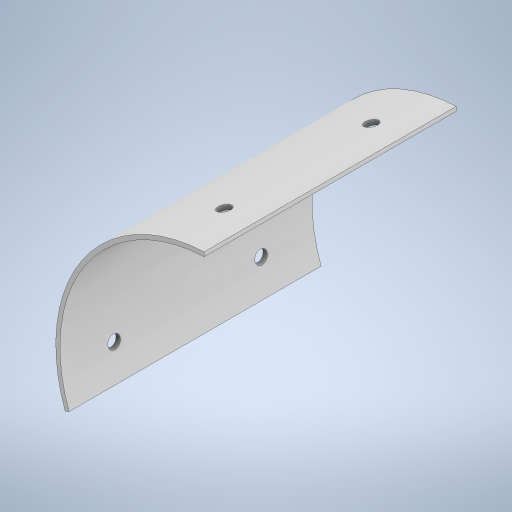
# Autodesk Inventor part: Electronics Door
Saved by Autodesk Inventor 2024 (Build 280153000, 153)
## iProperties
Created: 2024-04-23
Part Number: Electronics Door
Material: Generic
Document SubType Name: Modeling
Designer: auror
Density: 1 g/cm^3
Appearance: Default
Author: auror
Autodesk Inventor part; units mm, degrees
ref_plane "YZ Plane" through (0, 0, 0) normal (1, 0, 0) x (0, 1, 0)
ref_plane "XZ Plane" through (0, 0, 0) normal (0, 1, 0) x (-1, 0, 0)
ref_plane "XY Plane" through (0, 0, 0) normal (0, 0, 1) x (1, 0, 0)
sketch "Sketch1" plane through (0, 0, 0) normal (0, 0, 1) x (1, 0, 0)
  line L0 (0, 39.5237) -> (0, -43.4686) construction
  line L1 (-45.3066, 0) -> (2.8066, 0) construction
  line L2 (-11.1644, 34.052) -> (-34, 0) construction
  line L3 (2.8066, 0) -> (-40.0076, 0) construction
  line L4 (16.398, -33.1268) -> (-15.7593, 45.2513) construction
  line L5 (2.8066, 0) -> (-40.7672, -15.8596) construction
  arc A0 (-10.7848, 33.1268) -> (-33, 0) centre (2.8066, 0) ccw
  arc A1 (-11.1644, 34.052) -> (-34, 0) centre (2.8066, 0) ccw
  line L6 (1.3246, 36.7767) -> (1.3246, 35.7759)
  line L7 (-33, 0) -> (-34, 0)
  arc A2 (1.3246, 35.7759) -> (-10.7848, 33.1268) centre (2.8066, 0) ccw
  arc A3 (-33, 0) -> (-30.8406, -12.2466) centre (2.8066, 0) ccw
  arc A4 (1.3246, 36.7767) -> (-11.1644, 34.052) centre (2.8066, 0) ccw
  arc A5 (-34, 0) -> (-31.7803, -12.5886) centre (2.8066, 0) ccw
  line L8 (-34, 0) -> (-33, 0) construction
  line L9 (-31.7803, -12.5886) -> (-30.8406, -12.2466)
  line L10 (-34, 0) -> (-33, 0)
  line L11 (-11.1644, 34.052) -> (-10.7848, 33.1268)
  line L12 (2.8066, 0) -> (0.7848, 50.1716) construction
  point P0 (0, 0)
  point P1 (0, 35.5701)
  point P2 (-35.7519, 0.9163)
  dimension "d17" = 41
  dimension "d18" = 0
  dimension "d19" = 0
  dimension "d22" = 20
  dimension "d26" = 0
  dimension "d27" = 0
  dimension "d28" = 0
  dimension "d29" = 0
  dimension "d73" = 0
  dimension "d74" = 20
  constraints: 26 end point, 14 point on circle, 11 point on line, 6 centre point, 4 coincident, 4 collinear, 3 vertical, 1 horizontal, 1 perpendicular
  measures "d17" distance of L2.start L2.end
  measures "d18" distance from line of L1 L2.end
  measures "d19" distance from line of L2.end L3
  measures "d22" angle of L5 L1
  measures "d26" distance of L2.end L8.start
  measures "d27" distance of L7.start L8.end
  measures "d28" distance of L2.start L11.start
  measures "d29" distance of A0.start L11.end
  measures "d73" distance from line of L6.start L12
  measures "d74" angle of L12 L4
extrude "Extrusion2" add sketch "Sketch1" along normal blind 60 contours L11 A4 L6 A2
extrude "Extrusion3" add sketch "Sketch1" along normal blind 60 fills toward (-27.7211, 20.4722) open curves A1 L7 A0
extrude "Extrusion4" add sketch "Sketch1" along normal blind 60 contours A3 L9 A5 L7
ref_plane "Work Plane2" through (-11.1644, 34.052, 0) normal (-0.3795786, 0.9251595, 0) x (-0.9251595, -0.3795786, 0)
sketch "Sketch3" plane through (-11.1644, 34.052, 0) normal (-0.3795786, 0.9251595, 0) x (-0.9251595, -0.3795786, 0)
  line L0 (36.7767, 0) -> (-12.5886, 0) projected
  line L1 (-0.001, 0) -> (-0.001, 27.4188)
  point P0 (2.5965, 0)
  point P1 (-5.001, 12.5)
  dimension "d37" = 12.5
  dimension "d38" = 5
  constraints: 2 end point, 2 vertical, 1 point on line
  measures "d37" distance from line of L0 point (-5.001, 12.5)
  measures "d38" distance from line of L1 point (-5.001, 12.5)
hole "Hole1" at (-6.5377, 35.9502, 12.5) direction (0.3795786, -0.9251595, 0) diameter 2 end through all counterbore diameter 3 counterbore depth 10
sketch "Sketch4" plane through (-11.1644, 34.052, 0) normal (-0.3795786, 0.9251595, 0) x (-0.9251595, -0.3795786, 0)
  line L0 (36.7767, 60) -> (-12.5886, 60) projected
  line L1 (-0.0225, 60) -> (-0.0225, 43.6273)
  point P0 (2.5965, 0)
  point P1 (-5.0225, 47.5)
  dimension "d46" = 12.5
  dimension "d47" = 5
  constraints: 2 end point, 2 vertical, 1 point on line
  measures "d46" distance from line of L0 point (-5.022, 47.5)
  measures "d47" distance from line of L1 point (-5.022, 47.5)
hole "Hole2" at (-6.5178, 35.9584, 47.5) direction (0.3795786, -0.9251595, 0) diameter 2 end through all counterbore diameter 3 counterbore depth 10
ref_plane "Work Plane3" through (-34, 0, 0) normal (-1, 0, 0) x (0, -1, 0)
sketch "Sketch5" plane through (-34, 0, 0) normal (-1, 0, 0) x (0, -1, 0)
  line L0 (12.5886, 0) -> (-36.7767, 0) projected
  line L1 (0, 0) -> (0, 12.4269)
  point P0 (5, 12.5)
  dimension "d55" = 12.5
  dimension "d56" = 5
  constraints: 2 end point, 2 vertical
  measures "d55" distance from line of L0 point (5, 12.5)
  measures "d56" distance from line of L1 point (5, 12.5)
hole "Hole3" at (-34, -5, 12.5) direction (1, 0, 0) diameter 2 end through all counterbore diameter 3 counterbore depth 10
sketch "Sketch6" plane through (-34, 0, 0) normal (-1, 0, 0) x (0, -1, 0)
  line L0 (12.5886, 60) -> (-36.7767, 60) projected
  line L1 (0, 60) -> (0, 35.011)
  point P0 (0, 0)
  point P1 (5, 47.5)
  dimension "d64" = 5
  dimension "d65" = 12.5
  constraints: 2 end point, 2 vertical, 1 point on line
  measures "d64" distance from line of L1 point (5, 47.5)
  measures "d65" distance from line of L0 point (5, 47.5)
hole "Hole4" at (-34, -5, 47.5) direction (1, 0, 0) diameter 2 end through all counterbore diameter 3 counterbore depth 10
body "Solid1"
